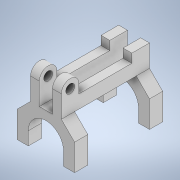
# Autodesk Inventor part: Assignment 2.4
Saved by Autodesk Inventor 2021.1 (Build 251245000, 245)
## iProperties
Created: 2021-05-14
Part Number: Assignment 2.4
Material: Generic
Document SubType Name: Modeling
Designer: as000166
Density: 1 g/cm^3
Appearance: Default
Author: as000166
Autodesk Inventor part; units mm, degrees
ref_plane "YZ Plane" through (0, 0, 0) normal (1, 0, 0) x (0, 1, 0)
ref_plane "XZ Plane" through (0, 0, 0) normal (0, 1, 0) x (-1, 0, 0)
ref_plane "XY Plane" through (0, 0, 0) normal (0, 0, 1) x (1, 0, 0)
sketch "Sketch1" plane through (0, 0, 0) normal (0, 0, 1) x (1, 0, 0)
  line L0 (0, 0) -> (44.45, 0)
  line L1 (44.45, 0) -> (44.45, 31.75)
  line L2 (44.45, 31.75) -> (31.75, 31.75)
  line L3 (31.75, 31.75) -> (31.75, 0)
  line L4 (0, 0) -> (0, 31.75)
  line L5 (0, 31.75) -> (12.7, 31.75)
  line L6 (12.7, 31.75) -> (12.7, 0)
  line L7 (63.5, -19.05) -> (44.45, 0)
  line L8 (-19.05, -19.05) -> (0, 0)
  line L9 (-19.05, -19.05) -> (-19.05, -57.15)
  line L10 (-19.05, -57.15) -> (0, -57.15)
  line L11 (0, -57.15) -> (63.5, -57.15)
  line L12 (63.5, -57.15) -> (63.5, -19.05)
  dimension "d0" = 44.45
  dimension "d1" = 31.75
  dimension "d2" = 12.7
  dimension "d3" = 31.75
  dimension "d4" = 12.7
  dimension "d9" = 38.1
  constraints: 26 end point, 7 perpendicular, 3 point on line, 1 horizontal, 1 vertical
  measures "d0" distance of L0.start L0.end
  measures "d1" distance of L0.end L1.end
  measures "d2" distance of L1.end L2.end
  measures "d3" distance of L0.start L4.end
  measures "d4" distance of L4.end L5.end
  measures "d9" distance of L8.start L9.end
extrude "Extrusion1" add sketch "Sketch1" against normal blind 127 contours L0 L7 L12 L11 L10 L9 L8
sketch "Sketch2" plane through (0, 0, 0) normal (0, 0, 1) x (1, 0, 0)
  line L0 (63.5, -57.15) -> (-19.05, -57.15) projected
  arc A0 (47.625, -38.1) -> (-3.175, -38.1) centre (22.225, -38.1) ccw
  line L1 (-3.175, -38.1) -> (-3.175, -57.15)
  line L2 (47.625, -38.1) -> (47.625, -57.15)
  point P0 (0, 0)
  dimension "d14" = 50.8
  constraints: 4 end point, 2 point on circle, 2 point on line, 1 centre point, 1 perpendicular, 1 vertical
  measures "d14" diameter of A0
extrude "Extrusion2" cut sketch "Sketch2" against normal blind 127
sketch "Sketch3" plane through (0, 0, 0) normal (0, 0, 1) x (1, 0, 0)
  line L0 (0, 0) -> (-19.05, -19.05) projected
  line L1 (0, 0) -> (0, 31.75)
  line L2 (0, 31.75) -> (12.7, 31.75)
  line L3 (12.7, 31.75) -> (12.7, 0)
  line L4 (44.45, 0) -> (0, 0) projected
  line L5 (44.45, 0) -> (44.45, 31.75)
  line L6 (44.45, 31.75) -> (31.75, 31.75)
  line L7 (31.75, 31.75) -> (31.75, 0)
  dimension "d17" = 31.75
  dimension "d18" = 12.7
  dimension "d19" = 31.75
  dimension "d20" = 12.7
  constraints: 12 end point, 3 perpendicular, 3 point on line, 1 vertical
  measures "d17" distance of L0.start L1.end
  measures "d18" distance of L1.end L2.end
  measures "d19" distance of L4.start L5.end
  measures "d20" distance of L5.end L6.end
extrude "Extrusion3" add sketch "Sketch3" against normal blind 127 contours L1 L2 L3 L4
sketch "Sketch4" plane through (0, 0, 0) normal (0, 0, 1) x (1, 0, 0)
  line L0 (12.7, 0) -> (44.45, 0) projected
  line L1 (44.45, 0) -> (44.45, 31.75)
  line L2 (44.45, 31.75) -> (31.75, 31.75)
  line L3 (31.75, 31.75) -> (31.75, 0)
  point P0 (0, 0)
  dimension "d23" = 31.75
  dimension "d24" = 12.7
  constraints: 6 end point, 2 perpendicular, 1 point on line, 1 vertical
  measures "d23" distance of L0.end L1.end
  measures "d24" distance of L1.end L2.end
extrude "Extrusion4" add sketch "Sketch4" against normal blind 127
sketch "Sketch5" plane through (63.5, -57.15, 0) normal (1, 0, 0) x (0, 0, -1)
  line L0 (107.95, 11.1125) -> (107.95, 57.15)
  line L1 (0, 57.15) -> (127, 57.15) projected
  line L2 (19.05, 10.2158) -> (19.05, 57.15)
  line L3 (107.95, 57.15) -> (19.05, 57.15)
  line L4 (19.05, 10.2158) -> (19.05, 0)
  line L5 (0, 0) -> (127, 0) projected
  line L6 (107.95, 11.1125) -> (107.95, 0)
  constraints: 10 end point, 6 point on line, 1 parallel, 1 perpendicular
extrude "Extrusion5" cut sketch "Sketch5" against normal blind 127
sketch "Sketch6" plane through (0, 0, 0) normal (0, 0, 1) x (1, 0, 0)
  line L0 (12.7, 31.75) -> (33.3375, 31.75)
  line L1 (31.75, 0) -> (31.75, 31.75) projected
  line L2 (33.3375, 31.75) -> (31.75, 0)
  line L3 (12.7, 0) -> (31.75, 0) projected
  line L4 (31.75, 0) -> (12.7, 0)
  line L5 (12.7, 31.75) -> (12.7, 0) projected
  line L6 (12.7, 0) -> (12.7, 31.75)
  point P0 (0, 0)
  constraints: 8 end point, 1 collinear, 1 horizontal, 1 perpendicular
extrude "Extrusion6" add sketch "Sketch6" against normal blind 127 contours L0 L1 L3 L5
sketch "Sketch7" plane through (44.45, 0, 0) normal (1, 0, 0) x (0, 0, -1)
  line L0 (0, 31.75) -> (127, 31.75) projected
  circle A0 centre (12.7, 31.75) radius 12.7
  point P0 (0, 0)
  point P1 (25.4, 31.75)
  dimension "d35" = 25.4
  constraints: 3 other
extrude "Extrusion7" add sketch "Sketch7" against normal blind 44.45 contours A0 L0 picked at (10.6191, 40.4828)
sketch "Sketch8" plane through (44.45, 0, -127) normal (1, 0, 0) x (0, 0, -1)
  circle A0 centre (-114.3, 31.75) radius 6.35
  point P0 (-127, 0)
  dimension "d39" = 12.7
  constraints: 1 centre point
  measures "d39" diameter of A0
extrude "Extrusion8" cut sketch "Sketch8" against normal blind 44.45
sketch "Sketch9" plane through (44.45, 0, -127) normal (1, 0, 0) x (0, 0, -1)
  line L0 (-101.6, 31.75) -> (0, 31.75) projected
  line L1 (-101.6, 31.75) -> (-101.6, 19.05)
  line L2 (-101.6, 19.05) -> (-25.4, 19.05)
  line L3 (-25.4, 19.05) -> (-25.4, 31.75)
  point P0 (-127, 0)
  dimension "d42" = 12.7
  constraints: 6 end point, 1 horizontal, 1 perpendicular, 1 point on line, 1 vertical
  measures "d42" distance of L0.start L1.end
extrude "Extrusion9" cut sketch "Sketch9" against normal through all
sketch "Sketch10" plane through (0, 0, 0) normal (0, 0, 1) x (1, 0, 0)
  line L0 (12.7, 0) -> (12.7, 44.45)
  line L1 (31.75, 0) -> (31.75, 44.45)
  line L2 (44.45, 44.45) -> (0, 44.45) projected
  line L3 (12.7, 44.45) -> (31.75, 44.45)
  line L4 (12.7, 0) -> (31.75, 0)
  line L5 (0, 0) -> (44.45, 0) projected
  dimension "d50" = 19.05
  constraints: 8 end point, 2 vertical, 1 collinear, 1 perpendicular, 1 point on line
  measures "d50" distance of L0.start L1.start
extrude "Extrusion10" cut sketch "Sketch10" against normal blind 127
body "Solid1"
